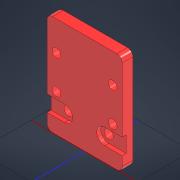
# Autodesk Inventor part: Camera-Base
Saved by Autodesk Inventor 2022.2 (Build 262287010, 287A)
## iProperties
Created: 2022-04-02
Part Number: Camera-Base
Material: ABS-Kunststoff
Document SubType Name: Modeling
Designer: sleib
Density: 1.06 g/cm^3
Appearance: Hellrot
Author: sleib
Autodesk Inventor part; units mm, degrees
ref_plane "YZ Plane" through (0, 0, 0) normal (1, 0, 0) x (0, 1, 0)
ref_plane "XZ Plane" through (0, 0, 0) normal (0, 1, 0) x (-1, 0, 0)
ref_plane "XY Plane" through (0, 0, 0) normal (0, 0, 1) x (1, 0, 0)
sketch "Skizze1" plane through (0, 0, 0) normal (0, 0, 1) x (1, 0, 0)
  line L0 (-14, -18.75) -> (14, -18.75)
  line L1 (14, -18.75) -> (14, 18.75)
  line L2 (14, 18.75) -> (-14, 18.75)
  line L3 (-14, 18.75) -> (-14, -18.75)
  line L4 (-14, -18.75) -> (14, 18.75) construction
  line L5 (14, -18.75) -> (-14, 18.75) construction
  circle A0 centre (-10.5, 7.75) radius 1.625
  circle A1 centre (-10.5, -4.75) radius 1.625
  circle A2 centre (10.5, -4.75) radius 1.625
  circle A3 centre (10.5, 7.75) radius 1.625
  line L6 (0, 18.75) -> (0, -18.75) construction
  line L7 (-14, -10.25) -> (14, -10.25) construction
  circle A4 centre (-7.5, -10.25) radius 1.7
  circle A5 centre (7.5, -10.25) radius 1.7
  circle A6 centre (-7.5, -10.25) radius 3
  circle A7 centre (7.5, -10.25) radius 3
  arc A8 (-12, 18.75) -> (-14, 16.75) centre (-12, 16.75) ccw
  arc A9 (14, 16.75) -> (12, 18.75) centre (12, 16.75) ccw
  line L8 (-7.5, -7.25) -> (-14, -7.25)
  line L9 (-7.5, -13.25) -> (-14, -13.25)
  line L10 (-14, -13.25) -> (-14, -7.25)
  line L11 (7.5, -7.25) -> (14, -7.25)
  line L12 (7.5, -13.25) -> (14, -13.25)
  line L13 (14, -13.25) -> (14, -7.25)
  line L14 (-10, -18.75) -> (7, -18.75)
  arc A10 (-14, -16.75) -> (-12, -18.75) centre (-12, -16.75) ccw
  arc A11 (12, -18.75) -> (14, -16.75) centre (12, -16.75) ccw
  point P0 (0, 0)
  point P1 (12.5, -1.6583)
  point P2 (-12.5, -1.6583)
  point P3 (12.5, 1.6583)
  point P4 (-12.5, 1.6583)
  dimension "d0" = 28
  dimension "d1" = 37.5
  dimension "d2" = 3.25
  dimension "d3" = 21
  dimension "d4" = 12.5
  dimension "d6" = 3.4
  dimension "d7" = 15
  dimension "d8" = 6
  dimension "d9" = 2
  dimension "d20" = 11
  dimension "d21" = 29
  dimension "d22" = 8.5
  constraints: 30 end point, 21 point on line, 12 centre point, 12 point on circle, 10 tangent, 8 equal radius, 5 midpoint, 3 perpendicular, 2 coincident, 2 collinear, 2 horizontal alignment, 2 parallel, 2 symmetric about line, 2 vertical alignment, 1 horizontal
  measures "d0" distance of L1.end L2.end
  measures "d1" distance of L2.end L0.start
  measures "d2" diameter of A0
  measures "d3" distance of A3.centre A0.centre
  measures "d4" distance of A1.centre A0.centre
  measures "d6" diameter of A4
  measures "d7" distance of A5.centre A4.centre
  measures "d8" diameter of A6
  measures "d9" radius of A8
  measures "d20" distance from line of A0.centre L2
  measures "d21" distance between parallel lines of L7 L2
  measures "d22" distance between parallel lines of L0 L7
extrude "Extrusion1" add sketch "Skizze1" against normal blind 4 contours A10 L3 L9 A6 L8 A8 L2 A9 L1 L11 A7 L12 A11 L0 | L3 L8 A6 L9 | A6 | L12 A7 L11 L1 | A7
extrude "Extrusion2" cut sketch "Skizze1" against normal blind 1.5 contours L3 L8 A6 L9 | A6 | L12 A7 L11 L1 | A7
